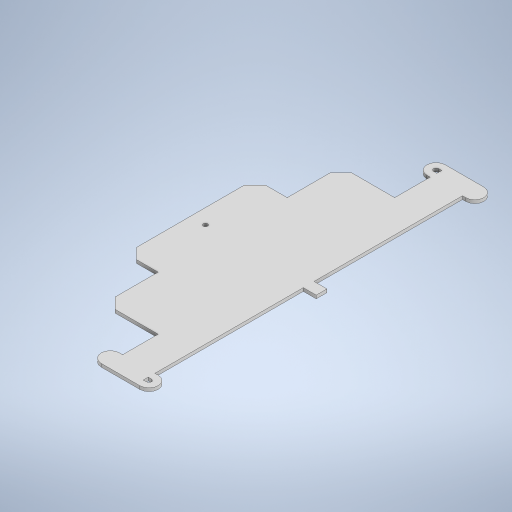
# Autodesk Inventor part: linefollower_chassy_model_3
Saved by Autodesk Inventor 2024 (Build 280153000, 153)
## iProperties
Created: 2024-02-27
Part Number: linefollower_chassy_model_3
Material: Generic
Document SubType Name: Modeling
Designer: kamil
Density: 1 g/cm^3
Appearance: Default
Author: kamil
Autodesk Inventor part; units mm, degrees
ref_plane "YZ Plane" through (0, 0, 0) normal (1, 0, 0) x (0, 1, 0)
ref_plane "XZ Plane" through (0, 0, 0) normal (0, 1, 0) x (-1, 0, 0)
ref_plane "XY Plane" through (0, 0, 0) normal (0, 0, 1) x (1, 0, 0)
sketch "Sketch1" plane through (0, 0, 0) normal (0, 1, 0) x (-1, 0, 0)
  line L0 (7.5, 80) -> (-7.5, 80)
  line L1 (-7.5, -80) -> (7.5, -80)
  line L2 (7.5, 75.75) -> (9, 75.75)
  line L3 (7.5, 80) -> (9, 80)
  line L4 (7.5, 71.5) -> (9, 71.5)
  arc A0 (9, 71.5) -> (9, 80) centre (9, 75.75) ccw
  line L5 (7.5, 74.6) -> (9, 74.6)
  line L6 (7.5, 76.9) -> (9, 76.9)
  arc A1 (9, 74.6) -> (9, 76.9) centre (9, 75.75) ccw
  line L7 (-7.5, 80) -> (-9, 80)
  line L8 (-7.5, 71.5) -> (-9, 71.5)
  arc A2 (-9, 80) -> (-9, 71.5) centre (-9, 75.75) ccw
  line L9 (-7.5, 74.6) -> (-9, 74.6)
  line L10 (-7.5, 76.9) -> (-9, 76.9)
  arc A3 (-9, 76.9) -> (-9, 74.6) centre (-9, 75.75) ccw
  line L11 (7.5, -80) -> (9, -80)
  line L12 (7.5, -71.5) -> (9, -71.5)
  arc A4 (9, -80) -> (9, -71.5) centre (9, -75.75) ccw
  line L13 (7.5, -74.6) -> (9, -74.6)
  line L14 (7.5, -76.9) -> (9, -76.9)
  arc A5 (9, -76.9) -> (9, -74.6) centre (9, -75.75) ccw
  arc A6 (-9, -71.5) -> (-9, -80) centre (-9, -75.75) ccw
  line L15 (-7.5, -71.5) -> (-9, -71.5)
  line L16 (-7.5, -74.6) -> (-9, -74.6)
  arc A7 (-9, -74.6) -> (-9, -76.9) centre (-9, -75.75) ccw
  line L17 (-7.5, -76.9) -> (-9, -76.9)
  line L18 (-7.5, -80) -> (-9, -80)
  line L19 (7.5, 55) -> (27.5, 55)
  line L20 (32.5, 50) -> (32.5, 30)
  line L21 (32.5, 30) -> (42.5, 30)
  line L22 (47.5, 25) -> (47.5, 0)
  line L23 (7.5, -55) -> (27.5, -55)
  line L24 (32.5, -50) -> (32.5, -30)
  line L25 (32.5, -30) -> (42.5, -30)
  line L26 (47.5, -25) -> (47.5, 0)
  line L27 (27.5, 55) -> (32.5, 50)
  line L28 (42.5, 30) -> (47.5, 25)
  line L29 (47.5, -25) -> (42.5, -30)
  line L30 (32.5, -50) -> (27.5, -55)
  circle A8 centre (40.5, 0) radius 1.025
  circle A9 centre (-11.5, 0) radius 1.025
  line L31 (-7.5, 2.5) -> (-13.5, 2.5)
  line L32 (-13.5, 2.5) -> (-13.5, -2.5)
  line L33 (-13.5, -2.5) -> (-7.5, -2.5)
  line L34 (-12.525, 0) -> (-13.5, 0) construction
  line L35 (7.5, 55) -> (7.5, 71.5)
  line L36 (7.5, 74.6) -> (7.5, 76.9)
  line L37 (-7.5, 76.9) -> (-7.5, 74.6)
  line L38 (-7.5, 71.5) -> (-7.5, 2.5)
  line L39 (7.5, -76.9) -> (7.5, -74.6)
  line L40 (7.5, -71.5) -> (7.5, -55)
  line L41 (-7.5, -2.5) -> (-7.5, -71.5)
  line L42 (-7.5, -74.6) -> (-7.5, -76.9)
  point P0 (8.25, 71.5)
  point P1 (32.5, 55)
  point P2 (47.5, 30)
  point P3 (32.5, -55)
  point P4 (47.5, -30)
  dimension "d26" = 2.05
  dimension "d0" = 160
  dimension "d2" = 1.5
  dimension "d3" = 4.25
  dimension "d5" = 4.25
  dimension "d6" = 4.25
  dimension "d7" = 1.15
  dimension "d8" = 1.15
  dimension "d9" = 1.15
  dimension "d10" = 25
  dimension "d11" = 25
  dimension "d12" = 15
  dimension "d13" = 25
  dimension "d14" = 25
  dimension "d15" = 5
  dimension "d16" = 5
  dimension "d17" = 5
  dimension "d18" = 5
  dimension "d19" = 5
  dimension "d20" = 5
  dimension "d21" = 5
  dimension "d22" = 5
  dimension "d24" = 2.05
  dimension "d25" = 7
  constraints: 86 end point, 18 parallel, 16 point on circle, 13 perpendicular, 9 centre point, 9 point on line, 8 horizontal, 5 coincident, 3 midpoint, 2 vertical, 1 horizontal alignment, 2 other
  measures "d0" distance of L1.end L0.start
  measures "d2" distance of L2.start L2.end
  measures "d3" distance between parallel lines of L0 L2
  measures "d5" distance from line of L2 point (8.25, 71.5)
  measures "d6" radius of A0
  measures "d7" distance between parallel lines of L5 L2
  measures "d8" distance between parallel lines of L2 L6
  measures "d9" radius of A1
  measures "d10" distance of L19.start point (32.5, 55)
  measures "d11" distance of point (32.5, 55) L20.end
  measures "d12" distance of L20.end point (47.5, 30)
  measures "d13" distance between parallel lines of L0 L19
  measures "d14" distance between parallel lines of L1 L23
  measures "d15" distance of L19.end point (32.5, 55)
  measures "d16" distance of L20.start point (32.5, 55)
  measures "d17" distance of L21.end point (47.5, 30)
  measures "d18" distance of L22.start point (47.5, 30)
  measures "d19" distance of L26.start point (47.5, -30)
  measures "d20" distance of L25.end point (47.5, -30)
  measures "d21" distance of L24.start point (32.5, -55)
  measures "d22" distance of L23.end point (32.5, -55)
  measures "d24" diameter of A8
  measures "d25" distance from line of A8.centre L26
extrude "Extrusion1" add sketch "Sketch1" along normal blind 1.5 contours L3 A0 L4 L35 L19 L27 L20 L21 L28 L22 L26 L29 L25 L24 L30 L23 L40 L12 A4 L11 L1 L18 A6 L15 L41 L33 L32 L31 L38 L8 A2 L7 L0 | L36 L6 A1 L5 | L42 L17 A7 L16 | A9
equation "\"d16\" = d15"
equation "\"d17\" = d15"
equation "\"d18\" = d17"
equation "\"d19\" = d15"
equation "\"d20\" = d19"
equation "\"d21\" = d15"
equation "\"d22\" = d21"
body "Solid1"
